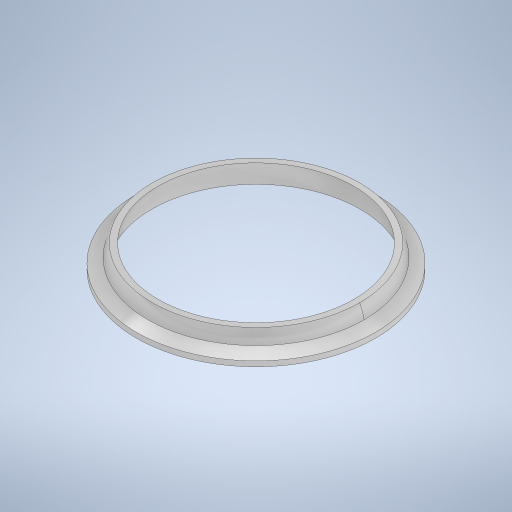
# Autodesk Inventor part: PMT_housing_ring
Saved by Autodesk Inventor 2023 (Build 270158000, 158)
## iProperties
Created: 2022-05-16
Part Number: PMT_housing_ring
Material: PVC, Unplasticized
Document SubType Name: Modeling
Designer: 50255
Density: 1.29 g/cm^3
Appearance: Aluminum - Dark
Author: 50255
Autodesk Inventor part; units mm, degrees
ref_plane "YZ Plane" through (0, 0, 0) normal (1, 0, 0) x (0, 1, 0)
ref_plane "XZ Plane" through (0, 0, 0) normal (0, 1, 0) x (-1, 0, 0)
ref_plane "XY Plane" through (0, 0, 0) normal (0, 0, 1) x (1, 0, 0)
sketch "Sketch1" plane through (0, 0, 0) normal (0, 0, 1) x (1, 0, 0)
  line L0 (0, 0) -> (25.6, 0)
  line L1 (0, 184.5) -> (101, 184.5) construction
  line L2 (0, 206.73) -> (95.0052, 206.73) construction
  ellipse E0 centre (0, 184.5) end of major axis (0, 250) minor radius 101 (101, 184.5) -> (95.0052, 206.73) ccw
  line L3 (95.0052, 206.73) -> (100.6517, 206.73)
  line L4 (101, 184.5) -> (101, 194.5) construction
  line L5 (101, 184.5) -> (106, 184.5)
  line L6 (0, 206.73) -> (0, 0)
  line L7 (101, 184.5) -> (116, 184.5)
  line L8 (116, 184.5) -> (116, 189.5)
  line L9 (116, 189.5) -> (104.9412, 194.5)
  spline S0 degree 5 poles (100.6517, 206.73) (101.8042, 204.4008) (102.8215, 202.0045) (103.6907, 199.5478) (104.4, 197.0418) (104.9412, 194.5) knots 0 0 0 0 0 0 1 1 1 1 1 1
  dimension "d16" = 95.0053
  dimension "d21" = 10
  dimension "d27" = 101
  dimension "d28" = 15
  dimension "d29" = 5
  constraints: 20 end point, 4 horizontal, 2 point on line, 1 perpendicular, 1 vertical, 8 other
  measures "d16" distance of L2.start L2.end
  measures "d21" distance of L1.end L4.end
  measures "d27" distance of L1.start L1.end
  measures "d28" distance of L1.end L7.end
  measures "d29" distance of L7.end L8.end
revolve "Revolution4" add sketch "Sketch1" angle 360 about axis through (0, 206.73, 0) along (0, -1, 0)
body "Solid4"
